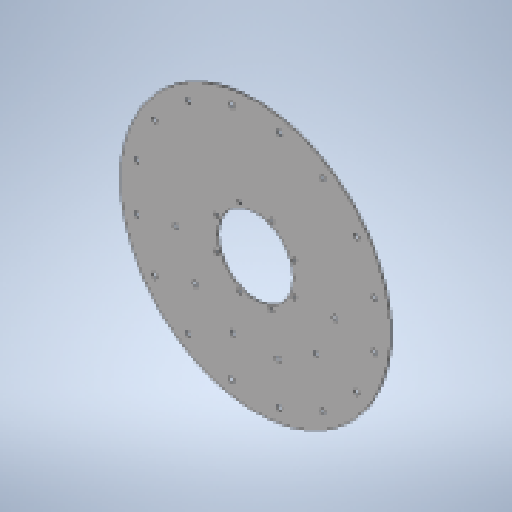
# Autodesk Inventor part: DMF 2.1 01 45 Gear ring 5
Saved by Autodesk Inventor 2026.2 (Build 302298000, 298)
## iProperties
Created: 2024-04-30
Part Number: DMF 2.1 01 45 Gear ring 5
Material: Generic
Document SubType Name: Sheet Metal
Designer: admin
Stock Number: Барабан_Сектор_Усилителя
Density: 1 g/cm^3
Sheet Metal Rule: Default
Sheet Metal Width: 500,000 mm
Sheet Metal Length: 500,000 mm
Sheet Metal Area: 250000,000 mm^2
Appearance: Default
Flat Pattern Width: 50 cm
Flat Pattern Length: 50 cm
Flat Pattern Area: 2500 cm^2
Author: pokla
Autodesk Inventor part; units mm, degrees
ref_plane "YZ Plane" through (0, 0, 0) normal (1, 0, 0) x (0, 1, 0)
ref_plane "XZ Plane" through (0, 0, 0) normal (0, 1, 0) x (-1, 0, 0)
ref_plane "XY Plane" through (0, 0, 0) normal (0, 0, 1) x (1, 0, 0)
sketch "Sketch1" plane through (0, 0, 0) normal (0, 0, 1) x (1, 0, 0)
  circle A0 centre (0, 0) radius 70
  circle A1 centre (0, 0) radius 250
  circle A2 centre (0, 0) radius 225 construction
  line L0 (-144.3376, -250) -> (-288.6751, 0) construction
  line L1 (-288.6751, 0) -> (-144.3376, 250) construction
  line L2 (-144.3376, 250) -> (144.3376, 250) construction
  line L3 (144.3376, 250) -> (288.6751, 0) construction
  line L4 (288.6751, 0) -> (144.3376, -250) construction
  line L5 (144.3376, -250) -> (-144.3376, -250) construction
  arc A3 (-28.3948, 223.2011) -> (-59.182, 217.0771) centre (0, 0) ccw construction
  arc A4 (-29.0131, 228.0619) -> (-60.4709, 221.8046) centre (0, 0) ccw construction
  arc A5 (-27.7764, 218.3403) -> (-57.8932, 212.3497) centre (0, 0) ccw construction
  arc A6 (-27.7764, 218.3403) -> (-29.0131, 228.0619) centre (-28.3948, 223.2011) ccw construction
  arc A7 (-60.4709, 221.8046) -> (-57.8932, 212.3497) centre (-59.182, 217.0771) ccw construction
  line L6 (-28.3948, 223.2011) -> (0, 0) construction
  line L7 (-59.182, 217.0771) -> (0, 0) construction
  line L8 (0, 0) -> (0, 70) construction
  line L9 (-43.8953, 220.6767) -> (0, 0) construction
  circle A8 centre (-43.8953, 220.6767) radius 4.9
  circle A9 centre (-125.0033, 187.0807) radius 4.9
  circle A10 centre (-187.0807, 125.0033) radius 4.9
  circle A11 centre (-220.6767, 43.8953) radius 4.9
  circle A12 centre (-220.6767, -43.8953) radius 4.9
  circle A13 centre (-187.0807, -125.0033) radius 4.9
  circle A14 centre (-125.0033, -187.0807) radius 4.9
  circle A15 centre (-43.8953, -220.6767) radius 4.9
  circle A16 centre (43.8953, -220.6767) radius 4.9
  circle A17 centre (125.0033, -187.0807) radius 4.9
  circle A18 centre (187.0807, -125.0033) radius 4.9
  circle A19 centre (220.6767, -43.8953) radius 4.9
  circle A20 centre (220.6767, 43.8953) radius 4.9
  circle A21 centre (187.0807, 125.0033) radius 4.9
  circle A22 centre (125.0033, 187.0807) radius 4.9
  circle A23 centre (43.8953, 220.6767) radius 4.9
  circle A24 centre (-147.7212, -26.0472) radius 4.9
  circle A25 centre (0, 0) radius 150 construction
  line L10 (0, 0) -> (-250, 0) construction
  line L11 (-147.7212, -26.0472) -> (0, 0) construction
  circle A26 centre (-111.4717, -100.3696) radius 4.9
  circle A27 centre (-41.3456, -144.1893) radius 4.9
  circle A28 centre (41.3456, -144.1893) radius 4.9
  circle A29 centre (111.4717, -100.3696) radius 4.9
  circle A30 centre (147.7212, -26.0472) radius 4.9
  circle A31 centre (29.658, 71.6007) radius 3.5
  line L12 (29.658, 71.6007) -> (0, 0) construction
  circle A32 centre (0, 0) radius 77.5 construction
  circle A33 centre (-29.658, 71.6007) radius 3.5
  circle A34 centre (-71.6007, 29.658) radius 3.5
  circle A35 centre (-71.6007, -29.658) radius 3.5
  circle A36 centre (-29.658, -71.6007) radius 3.5
  circle A37 centre (29.658, -71.6007) radius 3.5
  circle A38 centre (71.6007, -29.658) radius 3.5
  circle A39 centre (71.6007, 29.658) radius 3.5
  point P0 (0, -250)
  point P1 (216.5064, 125)
  point P2 (-216.5064, 125)
  dimension "d32" = 140
  dimension "d39" = 450
  dimension "d84" = 300
  dimension "d97" = 155
  dimension "d31" = 500
  dimension "d57" = 8
  dimension "d58" = 11.25
  dimension "d82" = 360
  dimension "d89" = 10
  dimension "d92" = 160
  dimension "d94" = 9.8
  dimension "d95" = 7
  dimension "d96" = 22.5
  dimension "d100" = 360
  measures "d31" diameter of A1
  measures "d57" angle of L7 L6
  measures "d58" angle of L8 L9
  measures "d89" angle of L11 L10
  measures "d94" diameter of A8
  measures "d95" diameter of A31
  measures "d96" angle of L12 L8
extrude "Plate4" add sketch "Sketch1" along normal blind 2
sketch "Sketch5" plane through (0, 0, 2) normal (0, 0, 1) x (1, 0, 0)
  line L0 (-1.6, -169) -> (1.6, -169)
  line L1 (1.6, -169) -> (1.6, -209)
  line L2 (1.6, -209) -> (-1.6, -209)
  line L3 (-1.6, -209) -> (-1.6, -169)
  line L4 (-207, -40) -> (-167, -40)
  line L5 (-167, -40) -> (-167, -43.2)
  line L6 (-167, -43.2) -> (-207, -43.2)
  line L7 (-207, -43.2) -> (-207, -40)
  line L8 (0, 0) -> (0, -169)
  line L9 (167, -40) -> (207, -40)
  line L10 (207, -40) -> (207, -43.2)
  line L11 (207, -43.2) -> (167, -43.2)
  line L12 (167, -43.2) -> (167, -40)
  dimension "d74" = 3.2
  dimension "d75" = 40
  dimension "d76" = 40
  dimension "d77" = 40
  dimension "d78" = 167
  dimension "d79" = 169
  constraints: 26 end point, 6 parallel, 3 equal length, 3 horizontal, 3 perpendicular, 1 collinear, 1 midpoint, 1 vertical, 1 other
  measures "d74" distance of L0.start L0.end
  measures "d75" distance of L0.end L1.end
  measures "d76" distance of L4.start L4.end
  measures "d77" distance from line of L8.start L4
  measures "d78" distance between parallel lines of L8 L5
  measures "d79" distance from line of L0 L8.start
feature "Mark1" [suppressed]
equation "\"d63\" = Thickness"
equation "\"BendRadius\" = Thickness"
equation "\"BendReliefWidth\" = Thickness"
equation "\"BendReliefDepth\" = 0.5 * Thickness"
equation "\"CornerReliefSize\" = 4 * Thickness"
equation "\"MinimumRemnant\" = 2 * Thickness"
equation "\"TransitionRadius\" = BendRadius"
equation "\"JacobiRadiusSize\" = BendRadius"
equation "\"GapSize\" = Thickness"
equation "\"Thickness\" = 2"
body "Solid3"
